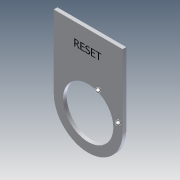
# Autodesk Inventor part: Reset Button Lable
Saved by Autodesk Inventor 2016 (Build 200138000, 138)
## iProperties
Created: 2005-06-20
Part Number: Reset Button Lable
Checked By: ~
Material: Generic
Document SubType Name: Modeling
Designer: BassBW
Manufacturer: Standard
Standards Organization: Custom
Density: 1 g/cm^3
Appearance: White
SCALE: 1:1
STOCK SIZE: SEE DWG
UNITS: ANSI
COMMODITY: MFG
Author: BassBW
Autodesk Inventor part; units mm, degrees
ref_plane "YZ Plane" through (0, 0, 0) normal (1, 0, 0) x (0, 1, 0)
ref_plane "XZ Plane" through (0, 0, 0) normal (0, 1, 0) x (-1, 0, 0)
ref_plane "XY Plane" through (0, 0, 0) normal (0, 0, 1) x (1, 0, 0)
sketch "Sketch1" plane through (0, 0, 0) normal (0, 0, 1) x (1, 0, 0)
  line L0 (30.1625, 0) -> (30.1625, 31.75)
  line L1 (30.1625, 31.75) -> (0, 31.75)
  line L2 (0, 31.75) -> (0, 0)
  arc A0 (0, 0) -> (30.1625, 0) centre (15.0813, 0) ccw
  dimension "d34" = 30.1625
  dimension "d35" = 31.75
  constraints: 6 end point, 2 point on circle, 2 tangent, 1 centre point, 1 horizontal, 1 parallel, 1 vertical
  measures "d34" distance of L0.end L1.end
  measures "d35" distance from line of A0.centre L1
extrude "Extrusion6" add sketch "Sketch1" along normal blind 1.5875
sketch "Sketch9" plane through (0, 0, 1.5875) normal (0, 0, 1) x (1, 0, 0)
  arc A0 (0, 0) -> (30.1625, 0) centre (15.0813, 0) ccw projected
  circle A1 centre (15.0813, 0) radius 11
  dimension "d38" = 22
  constraints: 1 centre point, 1 coincident
  measures "d38" diameter of A1
extrude "Extrusion7" cut sketch "Sketch9" against normal through all
sketch "Sketch10" plane through (0, 0, 1.5875) normal (0, 0, 1) x (1, 0, 0)
  line L0 (8.7312, 25.4) -> (21.4312, 25.4) construction
  line L1 (21.4312, 25.4) -> (21.4312, 22.225) construction
  line L2 (21.4312, 22.225) -> (8.7312, 22.225) construction
  line L3 (8.7312, 22.225) -> (8.7312, 25.4) construction
  circle A0 centre (15.0813, 0) radius 11 projected
  line L4 (11.3989, 22.2977) -> (10.8728, 22.2977)
  line L5 (10.8728, 22.2977) -> (9.9094, 23.5104)
  line L6 (9.9094, 23.5104) -> (9.4451, 23.5104)
  line L7 (9.4451, 23.5104) -> (9.4451, 22.2977)
  line L8 (9.4451, 22.2977) -> (9.04, 22.2977)
  line L9 (9.04, 22.2977) -> (9.04, 25.3457)
  line L10 (9.04, 25.3457) -> (9.8255, 25.3457)
  spline S0 degree 3 poles (9.8255, 25.3457) (10.0873, 25.3457) (10.4405, 25.2888) (10.6011, 25.1851) knots 0 0 0 0 1 1 1 1
  spline S1 degree 3 poles (10.6011, 25.1851) (10.7616, 25.0814) (10.9469, 24.7578) (10.9469, 24.5182) knots 0 0 0 0 1 1 1 1
  spline S2 degree 3 poles (10.9469, 24.5182) (10.9469, 24.1848) (10.606, 23.7327) (10.3145, 23.6241) knots 0 0 0 0 1 1 1 1
  line L11 (10.3145, 23.6241) -> (11.3989, 22.2977)
  spline S3 degree 3 poles (10.5245, 24.4861) (10.5245, 24.6195) (10.4306, 24.8245) (10.3318, 24.8912) knots 0 0 0 0 1 1 1 1
  spline S4 degree 3 poles (10.3318, 24.8912) (10.2454, 24.948) (10.0157, 24.9949) (9.8477, 24.9949) knots 0 0 0 0 1 1 1 1
  line L12 (9.8477, 24.9949) -> (9.4451, 24.9949)
  line L13 (9.4451, 24.9949) -> (9.4451, 23.8488)
  line L14 (9.4451, 23.8488) -> (9.8008, 23.8488)
  spline S5 degree 3 poles (9.8008, 23.8488) (9.9761, 23.8488) (10.2553, 23.9106) (10.3516, 24.0069) knots 0 0 0 0 1 1 1 1
  spline S6 degree 3 poles (10.3516, 24.0069) (10.4405, 24.0909) (10.5245, 24.328) (10.5245, 24.4861) knots 0 0 0 0 1 1 1 1
  line L15 (11.6409, 22.2977) -> (11.6409, 25.3457)
  line L16 (11.6409, 25.3457) -> (13.5478, 25.3457)
  line L17 (13.5478, 25.3457) -> (13.5478, 24.985)
  line L18 (13.5478, 24.985) -> (12.046, 24.985)
  line L19 (12.046, 24.985) -> (12.046, 24.1502)
  line L20 (12.046, 24.1502) -> (13.4465, 24.1502)
  line L21 (13.4465, 24.1502) -> (13.4465, 23.7895)
  line L22 (13.4465, 23.7895) -> (12.046, 23.7895)
  line L23 (12.046, 23.7895) -> (12.046, 22.6583)
  line L24 (12.046, 22.6583) -> (13.5478, 22.6583)
  line L25 (13.5478, 22.6583) -> (13.5478, 22.2977)
  line L26 (13.5478, 22.2977) -> (11.6409, 22.2977)
  spline S7 degree 3 poles (14.8421, 22.2433) (14.5111, 22.2433) (14.0467, 22.3816) (13.8417, 22.4804) knots 0 0 0 0 1 1 1 1
  line L27 (13.8417, 22.4804) -> (13.8417, 22.9893)
  line L28 (13.8417, 22.9893) -> (13.8714, 22.9893)
  spline S8 degree 3 poles (13.8714, 22.9893) (14.0714, 22.8015) (14.5778, 22.5941) (14.8124, 22.5941) knots 0 0 0 0 1 1 1 1
  spline S9 degree 3 poles (14.8124, 22.5941) (15.1484, 22.5941) (15.4917, 22.8732) (15.4917, 23.1029) knots 0 0 0 0 1 1 1 1
  spline S10 degree 3 poles (15.4917, 23.1029) (15.4917, 23.2857) (15.3114, 23.5129) (15.1162, 23.5697) knots 0 0 0 0 1 1 1 1
  spline S11 degree 3 poles (15.1162, 23.5697) (14.9755, 23.6092) (14.7408, 23.6636) (14.5654, 23.708) knots 0 0 0 0 1 1 1 1
  spline S12 degree 3 poles (14.5654, 23.708) (14.4073, 23.75) (14.1579, 23.876) (14.0615, 23.9773) knots 0 0 0 0 1 1 1 1
  spline S13 degree 3 poles (14.0615, 23.9773) (13.9677, 24.0785) (13.8639, 24.3502) (13.8639, 24.5281) knots 0 0 0 0 1 1 1 1
  spline S14 degree 3 poles (13.8639, 24.5281) (13.8639, 24.8986) (14.4419, 25.4) (14.889, 25.4) knots 0 0 0 0 1 1 1 1
  spline S15 degree 3 poles (14.889, 25.4) (15.1459, 25.4) (15.6004, 25.2987) (15.7955, 25.2024) knots 0 0 0 0 1 1 1 1
  line L29 (15.7955, 25.2024) -> (15.7955, 24.7183)
  line L30 (15.7955, 24.7183) -> (15.7659, 24.7183)
  spline S16 degree 3 poles (15.7659, 24.7183) (15.6201, 24.8517) (15.1656, 25.0493) (14.9162, 25.0493) knots 0 0 0 0 1 1 1 1
  spline S17 degree 3 poles (14.9162, 25.0493) (14.6346, 25.0493) (14.2863, 24.785) (14.2863, 24.5701) knots 0 0 0 0 1 1 1 1
  spline S18 degree 3 poles (14.2863, 24.5701) (14.2863, 24.3774) (14.4913, 24.1477) (14.684, 24.0958) knots 0 0 0 0 1 1 1 1
  spline S19 degree 3 poles (14.684, 24.0958) (14.8124, 24.0613) (15.1854, 23.9723) (15.3089, 23.9353) knots 0 0 0 0 1 1 1 1
  spline S20 degree 3 poles (15.3089, 23.9353) (15.6226, 23.8389) (15.9141, 23.4512) (15.9141, 23.1671) knots 0 0 0 0 1 1 1 1
  spline S21 degree 3 poles (15.9141, 23.1671) (15.9141, 22.9868) (15.7683, 22.641) (15.6374, 22.52) knots 0 0 0 0 1 1 1 1
  spline S22 degree 3 poles (15.6374, 22.52) (15.4917, 22.3866) (15.1212, 22.2433) (14.8421, 22.2433) knots 0 0 0 0 1 1 1 1
  line L31 (16.3265, 22.2977) -> (16.3265, 25.3457)
  line L32 (16.3265, 25.3457) -> (18.2334, 25.3457)
  line L33 (18.2334, 25.3457) -> (18.2334, 24.985)
  line L34 (18.2334, 24.985) -> (16.7316, 24.985)
  line L35 (16.7316, 24.985) -> (16.7316, 24.1502)
  line L36 (16.7316, 24.1502) -> (18.1321, 24.1502)
  line L37 (18.1321, 24.1502) -> (18.1321, 23.7895)
  line L38 (18.1321, 23.7895) -> (16.7316, 23.7895)
  line L39 (16.7316, 23.7895) -> (16.7316, 22.6583)
  line L40 (16.7316, 22.6583) -> (18.2334, 22.6583)
  line L41 (18.2334, 22.6583) -> (18.2334, 22.2977)
  line L42 (18.2334, 22.2977) -> (16.3265, 22.2977)
  line L43 (19.3894, 22.2977) -> (19.3894, 24.985)
  line L44 (19.3894, 24.985) -> (18.3668, 24.985)
  line L45 (18.3668, 24.985) -> (18.3668, 25.3457)
  line L46 (18.3668, 25.3457) -> (20.817, 25.3457)
  line L47 (20.817, 25.3457) -> (20.817, 24.985)
  line L48 (20.817, 24.985) -> (19.7945, 24.985)
  line L49 (19.7945, 24.985) -> (19.7945, 22.2977)
  line L50 (19.7945, 22.2977) -> (19.3894, 22.2977)
  dimension "d41" = 3.175
  dimension "d42" = 12.7
  dimension "d43" = 22.225
  dimension "d44" = 6.35
  constraints: 2 other
  measures "d41" distance between parallel lines of L0 L2
  measures "d42" distance between parallel lines of L1 L3
  measures "d43" distance from line of A0.centre L2
  measures "d44" distance from line of A0.centre L3
emboss "Emboss2" sketch "Sketch10" operation cut depth 0.1778 direction (0, 0, -1) contours L4 L5 L6 L7 L8 L9 L10 S0 S1 S2 L11 | L15 L16 L17 L18 L19 L20 L21 L22 L23 L24 L25 L26 | S7 L27 L28 S8 S9 S10 S11 S12 S13 S14 S15 L29 L30 S16 S17 S18 S19 S20 S21 S22 | L31 L32 L33 L34 L35 L36 L37 L38 L39 L40 L41 L42 | L43 L44 L45 L46 L47 L48 L49 L50
equation "\"d44\" = 0.5 * d42"
body "Solid1"
